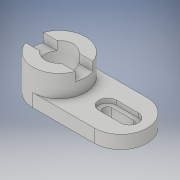
# Autodesk Inventor part: 複習一
Saved by Autodesk Inventor 2017 (Build 210142000, 142)
## iProperties
Part Number: 複習一
Material: 一般
Document SubType Name: Modeling
Designer: user01
Density: 1 g/cm^3
Appearance: 預設
Author: user01
Autodesk Inventor part; units mm, degrees
ref_plane "YZ Plane" through (0, 0, 0) normal (1, 0, 0) x (0, 1, 0)
ref_plane "XZ Plane" through (0, 0, 0) normal (0, 1, 0) x (-1, 0, 0)
ref_plane "XY Plane" through (0, 0, 0) normal (0, 0, 1) x (1, 0, 0)
sketch "草圖1" plane through (0, 0, 0) normal (0, 1, 0) x (-1, 0, 0)
  circle A0 centre (0, 0) radius 30
  line L0 (0, -30) -> (-70, -30)
  arc A1 (-70, 30) -> (-70, -30) centre (-70, 0) ccw
  line L1 (0, 30) -> (-70, 30)
  dimension "d0" = 70
  dimension "d1" = 30
  dimension "d2" = 60
  constraints: 4 end point, 4 point on circle, 3 tangent, 2 centre point, 2 horizontal, 1 coincident
  measures "d0" distance of A1.centre point (0, 0)
  measures "d1" radius of A1
  measures "d2" diameter of A0
extrude "擠出1" add sketch "草圖1" along normal blind 15
sketch "草圖2" plane through (0, 15, 0) normal (0, 1, 0) x (1, 0, 0)
  arc A0 (0, 30) -> (0, -30) centre (0, 0) ccw projected
  line L0 (0, -30) -> (70, -30) projected
  arc A1 (70, -30) -> (70, 30) centre (70, 0) ccw projected
  line L1 (70, 30) -> (0, 30) projected
  circle A2 centre (0, 0) radius 30
  constraints: 1 coincident, 1 vertical alignment, 2 other
extrude "擠出2" add sketch "草圖2" along normal blind 25 contours A2 A0
sketch "草圖3" plane through (0, 40, 0) normal (0, 1, 0) x (1, 0, 0)
  circle A0 centre (0, 0) radius 16
  dimension "d7" = 32
  constraints: 1 centre point, 1 coincident
  measures "d7" diameter of A0
extrude "擠出3" cut sketch "草圖3" against normal up to next
sketch "草圖4" plane through (0, 40, 0) normal (0, 1, 0) x (1, 0, 0)
  line L0 (-34.5334, 10) -> (33.6388, 10)
  line L1 (33.6388, 10) -> (33.6388, -10)
  line L2 (33.6388, -10) -> (-34.5334, -10)
  line L3 (-34.5334, -10) -> (-34.5334, 10)
  line L4 (-29.5296, 0) -> (41.1192, 0)
  point P0 (0, 0)
  dimension "d10" = 20
  constraints: 10 end point, 3 perpendicular, 2 horizontal, 1 point on line, 1 other
  measures "d10" distance between parallel lines of L0 L2
extrude "擠出4" cut sketch "草圖4" against normal blind 10
sketch "草圖5" plane through (0, 15, 0) normal (0, 1, 0) x (1, 0, 0)
  line L0 (48.3987, 0) -> (103.2063, 0)
  line L1 (55, 10) -> (80, 10)
  line L2 (55, -10) -> (80, -10)
  arc A0 (80, -10) -> (80, 10) centre (80, 0) ccw
  arc A1 (55, 10) -> (55, -10) centre (55, 0) ccw
  line L3 (0, 0) -> (0, 8.9825) construction
  dimension "d13" = 55
  dimension "d14" = 25
  dimension "d15" = 10
  dimension "d16" = 10
  constraints: 8 end point, 6 point on circle, 5 point on line, 3 horizontal, 2 centre point, 2 tangent, 1 vertical
  measures "d13" distance from line of A1.centre L3
  measures "d14" distance of A0.centre A1.centre
  measures "d15" radius of A0
  measures "d16" radius of A1
extrude "擠出5" cut sketch "草圖5" against normal blind 5
sketch "草圖6" plane through (0, 10, 0) normal (0, 1, 0) x (1, 0, 0)
  line L0 (55, 5) -> (80, 5)
  arc A0 (55, 5) -> (55, -5) centre (55, 0) ccw
  arc A1 (80, -5) -> (80, 5) centre (80, 0) ccw
  line L1 (55, -5) -> (80, -5)
  line L2 (0, 0) -> (0, 5.5956) construction
  line L3 (0, 0) -> (10.788, 0) construction
  line L4 (0, -30) -> (70, -30) projected
  dimension "d19" = 55
  dimension "d20" = 25
  dimension "d22" = 5
  dimension "d23" = 5
  dimension "d25" = 30
  dimension "d26" = 0
  constraints: 8 end point, 4 point on circle, 3 tangent, 2 centre point, 2 horizontal, 1 vertical
  measures "d19" distance from line of A0.centre L2
  measures "d20" distance of A1.centre A0.centre
  measures "d22" radius of A0
  measures "d23" radius of A1
  measures "d25" distance from line of A0.centre L4
  measures "d26" angle of L1 L0
extrude "擠出6" cut sketch "草圖6" against normal blind 10
